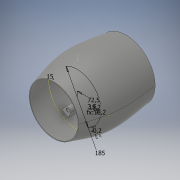
# Autodesk Inventor part: Form
Saved by Autodesk Inventor 2018.3 (Build 223284000, 284)
## iProperties
Created: 2018-07-22
Part Number: Form
Material: Generisch
Document SubType Name: Modeling
Designer: JochenAlt
Density: 1 g/cm^3
Appearance: Textur - grau
Author: JochenAlt
Autodesk Inventor part; units mm, degrees
ref_plane "YZ Plane" through (0, 0, 0) normal (1, 0, 0) x (0, 1, 0)
ref_plane "XZ Plane" through (0, 0, 0) normal (0, 1, 0) x (-1, 0, 0)
ref_plane "XY Plane" through (0, 0, 0) normal (0, 0, 1) x (1, 0, 0)
sketch "Skizze3" plane through (0, 0, 0) normal (0, 0, 1) x (1, 0, 0)
  line L0 (0, 295.492) -> (0, -259.2487) construction
  line L1 (-139.25, 0) -> (205.5, 0) construction
  line L2 (112.5, 190) -> (110, 190)
  circle A0 centre (0, 0) radius 90 construction
  circle A1 centre (0, -90) radius 90 construction
  line L3 (93, -90) -> (95.5, -90)
  line L4 (93, -90) -> (130.4373, 31.2709) construction
  line L5 (130.4373, 44.3072) -> (110, 190) construction
  spline S0 degree 3 poles (93, -90) (130.4373, 31.2709) (130.4373, 44.3072) (110, 190) knots 1 1 1 1 2 2 2 2
  line L6 (112.5, 190) -> (132.4373, 47.8716) construction
  line L7 (132.4373, 29.6513) -> (95.5, -90) construction
  spline S1 degree 3 poles (112.5, 190) (132.4373, 47.8716) (132.4373, 29.6513) (95.5, -90) knots 1 1 1 1 2 2 2 2
  line L8 (153.75, 101.6438) -> (156.25, 101.6438) construction
  line L9 (153.75, 101.6438) -> (156.25, 101.6438) construction
  line L10 (132.4373, 47.8716) -> (132.4373, 29.6513) construction
  line L11 (130.4373, 31.2709) -> (130.4373, 44.3072) construction
  line L12 (63.6396, 63.6396) -> (107.1267, 107.1267) construction
  line L13 (63.6396, -26.3604) -> (107.1267, 17.1267) construction
  circle A2 centre (107.1267, 17.1267) radius 8.5 construction
  circle A3 centre (107.1267, 107.1267) radius 8.5 construction
  line L14 (93, -90) -> (90, -90) construction
  line L15 (115.5316, 15.8592) -> (120.4757, 15.1136) construction
  line L16 (115.5801, 108.0154) -> (120.5527, 108.5381) construction
  line L17 (114.228, 136.6011) -> (117.2039, 136.9806) construction
  arc A4 (109.9551, 124.0972) -> (109.9551, 145.3104) centre (99.3485, 134.7038) ccw construction
  line L18 (109.9551, 145.3104) -> (55.3888, 199.8767) construction
  line L19 (109.9551, 124.0972) -> (65.9557, 80.0979) construction
  line L20 (112.5, 190) -> (109.5955, 210.7056) construction
  line L21 (109.5955, 210.7056) -> (102.5, 215) construction
  spline S2 degree 2 poles (112.5, 190) (109.5955, 210.7056) (102.5, 215) knots 1 1 1 2 2 2
  line L22 (110, 190) -> (107.0955, 210.7056) construction
  line L23 (107.0955, 210.7056) -> (100, 215) construction
  spline S3 degree 2 poles (110, 190) (107.0955, 210.7056) (100, 215) knots 1 1 1 2 2 2
  line L24 (102.5, 215) -> (100, 215)
  line L25 (110, 190) -> (110, 185)
  line L26 (110, 185) -> (108, 185)
  line L27 (108, 185) -> (108, 183)
  line L28 (108, 183) -> (110.9803, 183)
  line L29 (110, 190) -> (59.8, 190) construction
  line L30 (59.8, 190) -> (59.8, 185)
  line L31 (59.8, 185) -> (22, 172.5)
  arc A5 (49.9582, 183.7454) -> (59.8, 190) centre (42.4636, 206.409) ccw
  line L32 (49.9582, 183.7454) -> (22, 174.5)
  line L33 (22, 174.5) -> (22, 172.5)
  line L34 (59.8, 185) -> (108, 185) construction
  line L35 (22, 174.5) -> (9.0124, 174.5)
  line L36 (9.0124, 174.5) -> (9.0124, 172.5)
  line L37 (9.0124, 172.5) -> (22, 172.5)
  point P0 (90, 149.8145)
  point P1 (22, 173.5)
  dimension "d13" = 180
  dimension "d108" = 17
  dimension "d7" = 190
  dimension "d11" = 2.5
  dimension "d14" = 90
  dimension "d18" = 2.5
  dimension "d19" = 2.5
  dimension "d105" = 2
  dimension "d106" = 61.5
  dimension "d107" = 45
  dimension "d110" = 3
  dimension "d111" = 5
  dimension "d112" = 5
  dimension "d119" = 10
  dimension "d120" = 15
  dimension "d121" = 29
  dimension "d122" = 3
  dimension "d127" = 2.5
  dimension "d128" = 100
  dimension "d129" = 25
  dimension "d137" = 5
  dimension "d149" = 2
  dimension "d181" = 2
  dimension "d183" = 59.8
  dimension "d184" = 22
  dimension "d185" = 15.5
  constraints: 52 end point, 10 horizontal, 9 point on circle, 8 parallel, 5 point on line, 4 perpendicular, 3 centre point, 3 equal length, 3 tangent, 3 vertical, 2 coincident, 2 line through centre, 1 collinear, 1 midpoint, 31 other
  measures "d7" distance between parallel lines of L1 L2
  measures "d11" distance of L2.start L2.end
  measures "d14" distance of A1.centre point (0, 0)
  measures "d18" distance of L3.end L3.start
  measures "d19" distance of L8.start L8.end
  measures "d105" distance between parallel lines of L10 L11
  measures "d106" distance of L12.start L12.end
  measures "d107" angle of L0 L12
  measures "d110" distance of L3.start L14.end
  measures "d111" distance of L15.start L15.end
  measures "d112" distance of L16.start L16.end
  measures "d119" distance from line of L19.start L12
  measures "d120" radius of A4
  measures "d121" distance from line of L18 point (107.127, 107.127)
  measures "d122" distance of L17.start L17.end
  measures "d127" distance of L21.end L23.end
  measures "d128" distance from line of L0 L23.end
  measures "d129" distance between parallel lines of L2 L24
  measures "d137" distance of L2.end L25.end
  measures "d149" distance of L26.end L27.end
  measures "d181" distance of L31.end L32.end
  measures "d183" distance between parallel lines of L30 L0
  measures "d184" distance between parallel lines of L0 L33
  measures "d185" distance between parallel lines of L35 L29
revolve "Umdrehung1" add sketch "Skizze3" angle 360 about axis through (0, 0, 0) along (0, -1, 0) contours S1 L3 S0 L2 | S0 L28 L27 L26 L25
sketch "Skizze7" plane through (0, 0, 0) normal (0, 1, 0) x (-1, 0, 0)
  arc A0 (-91.4094, 14.1621) -> (-91.4094, -14.1621) centre (0, 0) ccw
  line L0 (-70.8006, -10.9691) -> (-91.4094, -14.1621)
  line L1 (-70.8006, 10.9691) -> (-91.4094, 14.1621)
  line L2 (-112.5, 0) -> (-125.8117, 0) construction
  arc A1 (-70.8006, -10.9691) -> (-70.8006, 10.9691) centre (-72.5, 0) ccw
  circle A2 centre (-72.5, 0) radius 6.6
  line L3 (-91.4094, -14.1621) -> (-108.7031, -16.8414)
  line L4 (-91.4094, 14.1621) -> (-108.7031, 16.8414)
  arc A3 (-54.9, 95.0896) -> (-54.9, -95.0896) centre (0, 0) ccw
  circle A4 centre (0, 0) radius 110 construction
  line L5 (0, -140) -> (0, 140) construction
  arc A5 (-106.5291, 16.5046) -> (-106.5291, -16.5046) centre (0, 0) ccw
  line L6 (-37.4, -64.7787) -> (-37.4, -64.7787)
  arc A6 (-93.1474, -14.114) -> (-93.1474, -14.114) centre (0.2914, 0.0441) ccw
  arc A7 (-74, -8.9755) -> (-71, -8.9755) centre (-72.5, 0) ccw
  arc A8 (-71, 8.9755) -> (-74, 8.9755) centre (-72.5, 0) ccw
  arc A9 (-71, -7.4505) -> (-71, 7.4505) centre (-72.5, 0) ccw
  arc A10 (-74, 7.4505) -> (-74, -7.4505) centre (-72.5, 0) ccw
  line L7 (-71, -8.9755) -> (-71, -7.4505)
  line L8 (-71, 7.4505) -> (-71, 8.9755)
  line L9 (-74, -8.9755) -> (-74, -7.4505)
  line L10 (-74, 7.4505) -> (-74, 8.9755)
  line L11 (-72.5, -9.1) -> (-72.5, 9.1) construction
  point P0 (-110, 0)
  point P1 (-95.5, 0)
  dimension "d32" = 185
  dimension "d116" = 0.2
  dimension "d142" = 72.5
  dimension "d192" = 15
  dimension "d194" = 2
  dimension "d196" = 15.2
  dimension "d197" = 1
  dimension "d199" = 3
  dimension "d200" = 18.2
  dimension "d201" = 3.5
  constraints: 22 point on circle, 20 end point, 10 centre point, 6 coincident, 5 vertical, 4 collinear, 4 point on line, 2 concentric, 2 tangent, 1 midpoint, 2 other
  measures "d32" diameter of A0
  measures "d116" radial gap between concentric circles of A4 A3
  measures "d142" distance of A1.centre point (0, 0)
  measures "d194" radial gap between concentric circles of A3 A5
  measures "d196" diameter of A9
  measures "d197" radial gap between concentric circles of A2 A9
  measures "d199" distance between parallel lines of L9 L7
  measures "d200" diameter of A7
  measures "d201" radial gap between concentric circles of A1 A9
extrude "Extrusion5" add sketch "Skizze7" along normal blind 30 separate body contours L1 A1 L0 A0
extrude "Extrusion8" add sketch "Skizze7" along normal blind 2 from surface at 0 contours L9 A10 L10 A8 L8 A9 L7 A7 bodies 2
pattern_circular "Runde Anordnung2" count 3 over 360 about axis through (0, -10, 0) along (0, 1, 0) bodies 2
equation "\"d14\" = 0.5 * d13"
equation "\"d18\" = d17"
equation "\"d16\" = d11"
equation "\"d17\" = d16"
